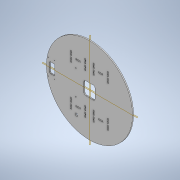
# Autodesk Inventor part: Нижний_круг_платформа
Saved by Autodesk Inventor 2020 (Build 240168000, 168)
## iProperties
Created: 2022-02-01
Part Number: Нижний_круг_платформа
Material: Типовые
Document SubType Name: Modeling
Designer: Администратор
Density: 1 g/cm^3
Appearance: По умолчанию
Autodesk Inventor part; units mm, degrees
ref_plane "XY Plane" through (0, 0, 0) normal (0, 0, 1) x (1, 0, 0)
sketch "0" plane through (0, 0, 0) normal (0, 0, 1) x (1, 0, 0)
  circle A0 centre (-79.9892, -71.9962) radius 3
  circle A1 centre (-79.9892, 72.0038) radius 3
  circle A2 centre (-237.2694, -46.8488) radius 1.6
  circle A3 centre (-237.2694, 48.1512) radius 1.6
  circle A4 centre (-204.2694, 48.1512) radius 1.6
  circle A5 centre (-204.2694, -46.8488) radius 1.6
  line L0 (-226.7694, -28.8488) -> (-206.7694, -28.8488)
  line L1 (-201.7694, -23.8488) -> (-201.7694, 25.1512)
  line L2 (-206.7694, 30.1512) -> (-226.7694, 30.1512)
  line L3 (-231.7694, 25.1512) -> (-231.7694, -23.8488)
  arc A6 (-201.7694, 25.1512) -> (-206.7694, 30.1512) centre (-206.7694, 25.1512) ccw
  arc A7 (-226.7694, 30.1512) -> (-231.7694, 25.1512) centre (-226.7694, 25.1512) ccw
  arc A8 (-231.7694, -23.8488) -> (-226.7694, -28.8488) centre (-226.7694, -23.8488) ccw
  arc A9 (-206.7694, -28.8488) -> (-201.7694, -23.8488) centre (-206.7694, -23.8488) ccw
  line L4 (32.5108, -27.4962) -> (32.5108, 27.5038)
  line L5 (-32.4892, 27.5038) -> (-32.4892, -27.4962)
  line L6 (110.0108, -121.9962) -> (110.0108, -131.9962)
  line L7 (110.0108, -131.9962) -> (104.0108, -131.9962)
  line L8 (104.0108, -131.9962) -> (104.0108, -121.9962)
  line L9 (104.0108, -121.9962) -> (110.0108, -121.9962)
  line L10 (110.0108, -137.9962) -> (110.0108, -147.9962)
  line L11 (110.0108, -147.9962) -> (104.0108, -147.9962)
  line L12 (104.0108, -147.9962) -> (104.0108, -137.9962)
  line L13 (104.0108, -137.9962) -> (110.0108, -137.9962)
  circle A10 centre (107.0108, -134.9962) radius 1.6
  line L14 (27.0108, -121.9962) -> (27.0108, -131.9962)
  line L15 (27.0108, -131.9962) -> (21.0108, -131.9962)
  line L16 (21.0108, -131.9962) -> (21.0108, -121.9962)
  line L17 (21.0108, -121.9962) -> (27.0108, -121.9962)
  line L18 (27.0108, -137.9962) -> (27.0108, -147.9962)
  line L19 (27.0108, -147.9962) -> (21.0108, -147.9962)
  line L20 (21.0108, -147.9962) -> (21.0108, -137.9962)
  line L21 (21.0108, -137.9962) -> (27.0108, -137.9962)
  circle A11 centre (24.0108, -134.9962) radius 1.6
  line L22 (104.0108, -113.9962) -> (104.0108, -103.9962)
  line L23 (104.0108, -103.9962) -> (110.0108, -103.9962)
  line L24 (110.0108, -103.9962) -> (110.0108, -113.9962)
  line L25 (110.0108, -113.9962) -> (104.0108, -113.9962)
  line L26 (104.0108, -97.9962) -> (104.0108, -87.9962)
  line L27 (104.0108, -87.9962) -> (110.0108, -87.9962)
  line L28 (110.0108, -87.9962) -> (110.0108, -97.9962)
  line L29 (110.0108, -97.9962) -> (104.0108, -97.9962)
  circle A12 centre (107.0108, -100.9962) radius 1.6
  line L30 (27.0108, -87.9962) -> (27.0108, -97.9962)
  line L31 (27.0108, -97.9962) -> (21.0108, -97.9962)
  line L32 (21.0108, -97.9962) -> (21.0108, -87.9962)
  line L33 (21.0108, -87.9962) -> (27.0108, -87.9962)
  line L34 (27.0108, -103.9962) -> (27.0108, -113.9962)
  line L35 (27.0108, -113.9962) -> (21.0108, -113.9962)
  line L36 (21.0108, -113.9962) -> (21.0108, -103.9962)
  line L37 (21.0108, -103.9962) -> (27.0108, -103.9962)
  circle A13 centre (24.0108, -100.9962) radius 1.6
  line L38 (52.5108, -120.9962) -> (52.5108, -114.9962)
  line L39 (78.5108, -114.9962) -> (78.5108, -120.9962)
  line L40 (78.5108, -120.9962) -> (52.5108, -120.9962)
  line L41 (52.5108, -114.9962) -> (78.5108, -114.9962)
  line L42 (-20.9892, -121.9962) -> (-20.9892, -131.9962)
  line L43 (-20.9892, -131.9962) -> (-26.9892, -131.9962)
  line L44 (-26.9892, -131.9962) -> (-26.9892, -121.9962)
  line L45 (-26.9892, -121.9962) -> (-20.9892, -121.9962)
  line L46 (-20.9892, -137.9962) -> (-20.9892, -147.9962)
  line L47 (-20.9892, -147.9962) -> (-26.9892, -147.9962)
  line L48 (-26.9892, -147.9962) -> (-26.9892, -137.9962)
  line L49 (-26.9892, -137.9962) -> (-20.9892, -137.9962)
  circle A14 centre (-23.9892, -134.9962) radius 1.6
  line L50 (-103.9892, -121.9962) -> (-103.9892, -131.9962)
  line L51 (-103.9892, -131.9962) -> (-109.9892, -131.9962)
  line L52 (-109.9892, -131.9962) -> (-109.9892, -121.9962)
  line L53 (-109.9892, -121.9962) -> (-103.9892, -121.9962)
  line L54 (-103.9892, -137.9962) -> (-103.9892, -147.9962)
  line L55 (-103.9892, -147.9962) -> (-109.9892, -147.9962)
  line L56 (-109.9892, -147.9962) -> (-109.9892, -137.9962)
  line L57 (-109.9892, -137.9962) -> (-103.9892, -137.9962)
  circle A15 centre (-106.9892, -134.9962) radius 1.6
  line L58 (-26.9892, -113.9962) -> (-26.9892, -103.9962)
  line L59 (-26.9892, -103.9962) -> (-20.9892, -103.9962)
  line L60 (-20.9892, -103.9962) -> (-20.9892, -113.9962)
  line L61 (-20.9892, -113.9962) -> (-26.9892, -113.9962)
  line L62 (-26.9892, -97.9962) -> (-26.9892, -87.9962)
  line L63 (-26.9892, -87.9962) -> (-20.9892, -87.9962)
  line L64 (-20.9892, -87.9962) -> (-20.9892, -97.9962)
  line L65 (-20.9892, -97.9962) -> (-26.9892, -97.9962)
  circle A16 centre (-23.9892, -100.9962) radius 1.6
  line L66 (-103.9892, -87.9962) -> (-103.9892, -97.9962)
  line L67 (-103.9892, -97.9962) -> (-109.9892, -97.9962)
  line L68 (-109.9892, -97.9962) -> (-109.9892, -87.9962)
  line L69 (-109.9892, -87.9962) -> (-103.9892, -87.9962)
  line L70 (-103.9892, -103.9962) -> (-103.9892, -113.9962)
  line L71 (-103.9892, -113.9962) -> (-109.9892, -113.9962)
  line L72 (-109.9892, -113.9962) -> (-109.9892, -103.9962)
  line L73 (-109.9892, -103.9962) -> (-103.9892, -103.9962)
  circle A17 centre (-106.9892, -100.9962) radius 1.6
  line L74 (-78.4892, -120.9962) -> (-78.4892, -114.9962)
  line L75 (-52.4892, -114.9962) -> (-52.4892, -120.9962)
  line L76 (-52.4892, -120.9962) -> (-78.4892, -120.9962)
  line L77 (-78.4892, -114.9962) -> (-52.4892, -114.9962)
  line L78 (110.0108, 122.0038) -> (110.0108, 132.0038)
  line L79 (110.0108, 132.0038) -> (104.0108, 132.0038)
  line L80 (104.0108, 132.0038) -> (104.0108, 122.0038)
  line L81 (104.0108, 122.0038) -> (110.0108, 122.0038)
  line L82 (110.0108, 138.0038) -> (110.0108, 148.0038)
  line L83 (110.0108, 148.0038) -> (104.0108, 148.0038)
  line L84 (104.0108, 148.0038) -> (104.0108, 138.0038)
  line L85 (104.0108, 138.0038) -> (110.0108, 138.0038)
  circle A18 centre (107.0108, 135.0038) radius 1.6
  line L86 (27.0108, 122.0038) -> (27.0108, 132.0038)
  line L87 (27.0108, 132.0038) -> (21.0108, 132.0038)
  line L88 (21.0108, 132.0038) -> (21.0108, 122.0038)
  line L89 (21.0108, 122.0038) -> (27.0108, 122.0038)
  line L90 (27.0108, 138.0038) -> (27.0108, 148.0038)
  line L91 (27.0108, 148.0038) -> (21.0108, 148.0038)
  line L92 (21.0108, 148.0038) -> (21.0108, 138.0038)
  line L93 (21.0108, 138.0038) -> (27.0108, 138.0038)
  circle A19 centre (24.0108, 135.0038) radius 1.6
  line L94 (104.0108, 114.0038) -> (104.0108, 104.0038)
  line L95 (104.0108, 104.0038) -> (110.0108, 104.0038)
  line L96 (110.0108, 104.0038) -> (110.0108, 114.0038)
  line L97 (110.0108, 114.0038) -> (104.0108, 114.0038)
  line L98 (104.0108, 98.0038) -> (104.0108, 88.0038)
  line L99 (104.0108, 88.0038) -> (110.0108, 88.0038)
  line L100 (110.0108, 88.0038) -> (110.0108, 98.0038)
  line L101 (110.0108, 98.0038) -> (104.0108, 98.0038)
  circle A20 centre (107.0108, 101.0038) radius 1.6
  line L102 (27.0108, 88.0038) -> (27.0108, 98.0038)
  line L103 (27.0108, 98.0038) -> (21.0108, 98.0038)
  line L104 (21.0108, 98.0038) -> (21.0108, 88.0038)
  line L105 (21.0108, 88.0038) -> (27.0108, 88.0038)
  line L106 (27.0108, 104.0038) -> (27.0108, 114.0038)
  line L107 (27.0108, 114.0038) -> (21.0108, 114.0038)
  line L108 (21.0108, 114.0038) -> (21.0108, 104.0038)
  line L109 (21.0108, 104.0038) -> (27.0108, 104.0038)
  circle A21 centre (24.0108, 101.0038) radius 1.6
  line L110 (52.5108, 121.0038) -> (52.5108, 115.0038)
  line L111 (78.5108, 115.0038) -> (78.5108, 121.0038)
  line L112 (78.5108, 121.0038) -> (52.5108, 121.0038)
  line L113 (52.5108, 115.0038) -> (78.5108, 115.0038)
  line L114 (-20.9892, 122.0038) -> (-20.9892, 132.0038)
  line L115 (-20.9892, 132.0038) -> (-26.9892, 132.0038)
  line L116 (-26.9892, 132.0038) -> (-26.9892, 122.0038)
  line L117 (-26.9892, 122.0038) -> (-20.9892, 122.0038)
  line L118 (-20.9892, 138.0038) -> (-20.9892, 148.0038)
  line L119 (-20.9892, 148.0038) -> (-26.9892, 148.0038)
  line L120 (-26.9892, 148.0038) -> (-26.9892, 138.0038)
  line L121 (-26.9892, 138.0038) -> (-20.9892, 138.0038)
  circle A22 centre (-23.9892, 135.0038) radius 1.6
  line L122 (-103.9892, 122.0038) -> (-103.9892, 132.0038)
  line L123 (-103.9892, 132.0038) -> (-109.9892, 132.0038)
  line L124 (-109.9892, 132.0038) -> (-109.9892, 122.0038)
  line L125 (-109.9892, 122.0038) -> (-103.9892, 122.0038)
  line L126 (-103.9892, 138.0038) -> (-103.9892, 148.0038)
  line L127 (-103.9892, 148.0038) -> (-109.9892, 148.0038)
  line L128 (-109.9892, 148.0038) -> (-109.9892, 138.0038)
  line L129 (-109.9892, 138.0038) -> (-103.9892, 138.0038)
  circle A23 centre (-106.9892, 135.0038) radius 1.6
  line L130 (-26.9892, 114.0038) -> (-26.9892, 104.0038)
  line L131 (-26.9892, 104.0038) -> (-20.9892, 104.0038)
  line L132 (-20.9892, 104.0038) -> (-20.9892, 114.0038)
  line L133 (-20.9892, 114.0038) -> (-26.9892, 114.0038)
  line L134 (-26.9892, 98.0038) -> (-26.9892, 88.0038)
  line L135 (-26.9892, 88.0038) -> (-20.9892, 88.0038)
  line L136 (-20.9892, 88.0038) -> (-20.9892, 98.0038)
  line L137 (-20.9892, 98.0038) -> (-26.9892, 98.0038)
  circle A24 centre (-23.9892, 101.0038) radius 1.6
  line L138 (-103.9892, 88.0038) -> (-103.9892, 98.0038)
  line L139 (-103.9892, 98.0038) -> (-109.9892, 98.0038)
  line L140 (-109.9892, 98.0038) -> (-109.9892, 88.0038)
  line L141 (-109.9892, 88.0038) -> (-103.9892, 88.0038)
  line L142 (-103.9892, 104.0038) -> (-103.9892, 114.0038)
  line L143 (-103.9892, 114.0038) -> (-109.9892, 114.0038)
  line L144 (-109.9892, 114.0038) -> (-109.9892, 104.0038)
  line L145 (-109.9892, 104.0038) -> (-103.9892, 104.0038)
  circle A25 centre (-106.9892, 101.0038) radius 1.6
  line L146 (-78.4892, 121.0038) -> (-78.4892, 115.0038)
  line L147 (-52.4892, 115.0038) -> (-52.4892, 121.0038)
  line L148 (-52.4892, 121.0038) -> (-78.4892, 121.0038)
  line L149 (-78.4892, 115.0038) -> (-52.4892, 115.0038)
  circle A26 centre (-79.9892, -71.9962) radius 3
  circle A27 centre (-79.9892, 72.0038) radius 3
  circle A28 centre (-79.9892, -71.9962) radius 3
  circle A29 centre (-79.9892, 72.0038) radius 3
  line L150 (22.5108, -37.4962) -> (-22.4892, -37.4962)
  line L151 (-22.4892, 37.5038) -> (22.5108, 37.5038)
  arc A30 (-32.4892, -27.4962) -> (-22.4892, -37.4962) centre (-22.4892, -27.4962) ccw
  arc A31 (-22.4892, 37.5038) -> (-32.4892, 27.5038) centre (-22.4892, 27.5038) ccw
  arc A32 (32.5108, 27.5038) -> (22.5108, 37.5038) centre (22.5108, 27.5038) ccw
  arc A33 (22.5108, -37.4962) -> (32.5108, -27.4962) centre (22.5108, -27.4962) ccw
  circle A34 centre (-74.9892, -159.9962) radius 7.925
  circle A35 centre (0.0108, 0.0038) radius 250
  point P0 (-226.7694, 30.1512)
  point P1 (-201.7694, 25.1512)
  point P2 (-201.7694, -23.8488)
  point P3 (-22.4892, 37.5038)
  point P4 (22.5108, 37.5038)
  point P5 (32.5108, 27.5038)
  point P6 (32.5108, -27.4962)
  point P7 (-32.4892, -27.4962)
  point P8 (-32.4892, 27.5038)
  constraints: 304 end point, 36 centre point, 16 point on circle
extrude "Выдавливание1" add sketch "0" along normal blind 6
